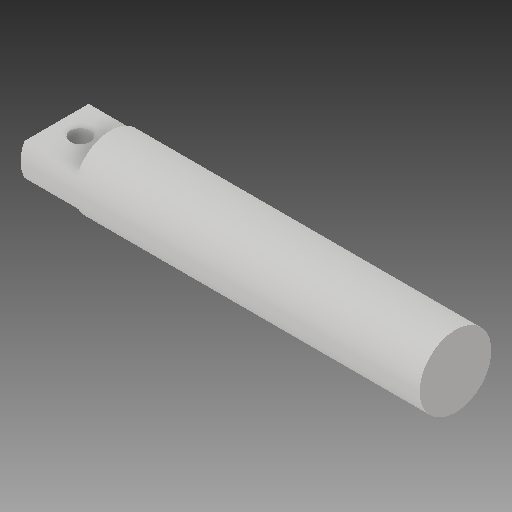
# Autodesk Inventor part: MSAL 32 50 Stand In
Saved by Autodesk Inventor 2019.4 (Build 234330000, 330)
## iProperties
Created: 2020-01-02
Part Number: MSAL 32 50 Stand In
Material: Generic
Document SubType Name: Modeling
Designer: Mark
Mass: 189.86 g
Surface Area: 245.839 cm^2
Volume: 189.86 cm^3
Density: 1 g/cm^3
Appearance: Default
Author: Mark
Autodesk Inventor part; units mm, degrees
ref_plane "YZ Plane" through (0, 0, 0) normal (1, 0, 0) x (0, 1, 0)
ref_plane "XZ Plane" through (0, 0, 0) normal (0, 1, 0) x (-1, 0, 0)
ref_plane "XY Plane" through (0, 0, 0) normal (0, 0, 1) x (1, 0, 0)
sketch "Sketch1" plane through (0, 0, 0) normal (1, 0, 0) x (0, 1, 0)
  circle A0 centre (0, 0) radius 18
  dimension "d0" = 36
  constraints: 1 centre point, 1 coincident
  measures "d0" diameter of A0
extrude "Extrusion1" add sketch "Sketch1" along normal blind 173
sketch "Sketch2" plane through (0, 0, 0) normal (-1, 0, 0) x (0, 0, 1)
  line L0 (20, -8) -> (-20, -8)
  line L1 (-20, -8) -> (-20, 8)
  line L2 (-20, 8) -> (20, 8)
  line L3 (20, 8) -> (20, -8)
  line L4 (20, -8) -> (-20, 8) construction
  line L5 (-20, -8) -> (20, 8) construction
  circle A0 centre (0, 0) radius 18 projected
  arc A1 (-16.1245, -8) -> (-17.098, -5.6266) centre (0, 0) ccw
  dimension "d3" = 40
  dimension "d5" = 16
  constraints: 12 end point, 4 point on circle, 2 concentric, 2 midpoint, 2 parallel, 1 centre point, 1 horizontal, 1 perpendicular, 1 point on line
  measures "d3" distance of L1.end L2.end
  measures "d5" distance between parallel lines of L0 L2
extrude "Extrusion2" add sketch "Sketch2" along normal blind 27 contours A0 L2 L0 | L0 L1 L2 A0 | A0 L2 L3 L0
sketch "Sketch3" plane through (-27, 0, 0) normal (-1, 0, 0) x (0, 0, 1)
  circle A0 centre (0, 0) radius 18
  circle A1 centre (0, 0) radius 50
  dimension "d8" = 36
  dimension "d9" = 100
  constraints: 2 centre point, 2 coincident
  measures "d8" diameter of A0
  measures "d9" diameter of A1
extrude "Extrusion3" cut sketch "Sketch3" against normal blind 27
sketch "Sketch4" plane through (0, 8, 16.1245) normal (0, 1, 0) x (1, 0, 0)
  circle A0 centre (-15, 16.1245) radius 5
  line L0 (-27, 0) -> (0, 0) projected
  line L1 (-27, 0) -> (-27, 32.249) projected
  point P0 (0, 16.1245)
  dimension "d12" = 10
  dimension "d13" = 16.1245
  dimension "d14" = 12
  constraints: 1 centre point
  measures "d12" diameter of A0
  measures "d13" distance from line of L0 A0.centre
  measures "d14" distance from line of L1 A0.centre
extrude "Extrusion4" cut sketch "Sketch4" against normal blind 16
body "Solid1"
